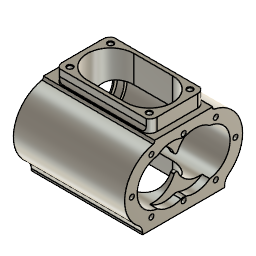
Body_ (Autodesk Fusion 360 design; units mm, degrees)
Autodesk Fusion 360 part; units mm, degrees
sketch "Sketch1" plane through (0, 0, 0) normal (1, 0, 0) x (0, 1, 0)
  circle A0 centre (-24, 0) radius 17.5
  arc A1 (-42.5, -37.3731) -> (-46.4362, -29.4214) centre (-52.5, -37.3731) ccw
  arc A2 (-31.4242, 36.2475) -> (-46.4362, -29.4214) centre (-24, 0) ccw
  arc A3 (-31.4242, 36.2475) -> (-30, 39.0239) centre (-31.8255, 38.2068) ccw
  line L0 (-30, 39.0239) -> (0, 39.0239)
  line L1 (0, 39.0239) -> (0, 0) construction
  line L2 (-42.5, -37.3731) -> (-42.5, -39.4214)
  line L3 (-42.5, -39.4214) -> (0, -39.4214)
  line L4 (0, 0) -> (0, -39.4214)
  line L5 (30, 39.0239) -> (0, 39.0239)
  arc A4 (30, 39.0239) -> (31.4242, 36.2475) centre (31.8255, 38.2068) ccw
  arc A5 (46.4362, -29.4214) -> (31.4242, 36.2475) centre (24, 0) ccw
  arc A6 (46.4362, -29.4214) -> (42.5, -37.3731) centre (52.5, -37.3731) ccw
  line L6 (42.5, -37.3731) -> (42.5, -39.4214)
  line L7 (42.5, -39.4214) -> (0, -39.4214)
  line L8 (0, 0) -> (0, -39.4214)
  circle A7 centre (24, 0) radius 17.5
  dimension "d1" = 35
  dimension "d2" = 24
  dimension "d3" = 2
  dimension "d4" = 37
  dimension "d5" = 10
  dimension "d6" = 10
  dimension "d7" = 42.5
  dimension "d8" = 30
  constraint horizontal L1.end A0.centre
  constraint tangent A1 A2
  constraint tangent A2 A3
  constraint horizontal L0
  constraint coincident L1.end L4.start
  constraint concentric A0 A2
  constraint vertical L2
  constraint perpendicular L2 L3
  constraint tangent A1 L2
  constraint vertical L4
  constraint vertical L1
  constraint symmetric A0 L1 A7
  constraint symmetric A1.start L1 A6.end
  constraint symmetric A1.end L1 A5.start
  constraint symmetric A1 L1 A6
  constraint symmetric A2.start L1 A4.end
  constraint symmetric A2 L1 A5
  constraint symmetric A3.end L1 L5.start
  constraint symmetric A3 L1 A4
  constraint symmetric L0.end L1 L5.end
  constraint symmetric L4.start L1 L8.start
  constraint symmetric L1 L2.end L6.end
  constraint symmetric L1 L3.end L4.end
  measures "d1" diameter of A0
  measures "d2" distance of L1.end A0.centre
  measures "d3" radius of A3
  measures "d4" radius of A2
  measures "d5" radius of A1
  measures "d6" vertical distance of A1.end L2.end
  measures "d7" distance of L2.end L3.end
  measures "d8" distance of A3.end L0.end
extrude "Extrude1" add sketch "Sketch1" along normal blind 115
sketch "Sketch2" plane through (115, 0, 0) normal (1, 0, 0) x (0, 1, 0)
  circle A0 centre (-24, 0) radius 17.5
  circle A1 centre (24, 0) radius 17.5
  arc A2 (46.4362, -29.4214) -> (31.4242, 36.2475) centre (24, 0) ccw
  arc A3 (30, 39.0239) -> (31.4242, 36.2475) centre (31.8255, 38.2068) ccw
  line L0 (30, 39.0239) -> (-30, 39.0239)
  arc A4 (-31.4242, 36.2475) -> (-30, 39.0239) centre (-31.8255, 38.2068) ccw
  arc A5 (-31.4242, 36.2475) -> (-46.4362, -29.4214) centre (-24, 0) ccw
  arc A6 (-42.5, -37.3731) -> (-46.4362, -29.4214) centre (-52.5, -37.3731) ccw
  line L1 (-42.5, -37.3731) -> (-42.5, -39.4214)
  line L2 (-42.5, -39.4214) -> (42.5, -39.4214)
  line L3 (42.5, -39.4214) -> (42.5, -37.3731)
  arc A7 (46.4362, -29.4214) -> (42.5, -37.3731) centre (52.5, -37.3731) ccw
  arc A8 (-1.8449, 9.2279) -> (1.8462, 9.2308) centre (0, 10) ccw
  arc A9 (1.8462, -9.2308) -> (-1.8461, -9.2308) centre (0, -10) ccw
  arc A10 (-1.8449, 9.2279) -> (-1.8461, -9.2308) centre (-24, 0) ccw
  arc A11 (1.8462, -9.2308) -> (1.8462, 9.2308) centre (24, 0) ccw
  dimension "d11" = 48
  dimension "d12" = 48
  dimension "d13" = 20
  dimension "d14" = 2
  dimension "d15" = 2
  constraint concentric A0 A10
  constraint concentric A1 A11
  constraint tangent A8 A11
  constraint tangent A9 A11
  measures "d11" diameter of A10
  measures "d12" diameter of A11
  measures "d13" vertical distance of A8.centre A9.centre
  measures "d14" radius of A9
  measures "d15" radius of A8
extrude "Extrude2" cut sketch "Sketch2" against normal blind 106.5 contours A8 A9 A10 A11
sketch "Sketch3" plane through (115, 0, 0) normal (1, 0, 0) x (0, 1, 0)
  arc A0 (1.8462, -9.2308) -> (-1.8461, -9.2308) centre (0, -10) ccw
  arc A1 (-1.8449, 9.2279) -> (-1.8461, -9.2308) centre (-24, 0) ccw
  arc A2 (-1.8449, 9.2279) -> (1.8462, 9.2308) centre (0, 10) ccw
  arc A3 (1.8462, -9.2308) -> (1.8462, 9.2308) centre (24, 0) ccw
  arc A4 (46.4362, -29.4214) -> (31.4242, 36.2475) centre (24, 0) ccw
  arc A5 (30, 39.0239) -> (31.4242, 36.2475) centre (31.8255, 38.2068) ccw
  line L0 (30, 39.0239) -> (-30, 39.0239)
  arc A6 (-31.4242, 36.2475) -> (-30, 39.0239) centre (-31.8255, 38.2068) ccw
  arc A7 (-31.4242, 36.2475) -> (-46.4362, -29.4214) centre (-24, 0) ccw
  arc A8 (-42.5, -37.3731) -> (-46.4362, -29.4214) centre (-52.5, -37.3731) ccw
  line L1 (-42.5, -37.3731) -> (-42.5, -39.4214)
  line L2 (-42.5, -39.4214) -> (42.5, -39.4214)
  line L3 (42.5, -39.4214) -> (42.5, -37.3731)
  arc A9 (46.4362, -29.4214) -> (42.5, -37.3731) centre (52.5, -37.3731) ccw
  line L4 (0, 0) -> (0, 67.4352) construction
  arc A10 (-2.5795, 27.2102) -> (-27, 23.8118) centre (-11.792, 3.9695) ccw
  arc A11 (-2.5795, 27.2102) -> (2.5795, 27.2102) centre (0, 33.7176) ccw
  arc A12 (27, 23.8118) -> (2.5795, 27.2102) centre (11.792, 3.9695) ccw
  dimension "d18" = 7
  dimension "d19" = 25
  dimension "d20" = 54
  constraint coincident L4.start origin
  constraint perpendicular L0 L4
  constraint coincident A1 A10.end
  constraint tangent A10 A11
  constraint tangent A11 A12
  constraint coincident A3 A12.start
  constraint equal A10 A12
  constraint symmetric L4 A10 A12
  constraint midpoint L4 A11.centre
  measures "d18" radius of A11
  measures "d19" radius of A10
  measures "d20" distance of A10.end A12.start
extrude "Extrude3" cut sketch "Sketch3" against normal blind 8 contours A1 A2 A3 A10 A11 A12
sketch "Sketch4" plane through (8.5, 0, 0) normal (1, 0, 0) x (0, 1, 0)
  circle A0 centre (-24, 0) radius 17.5
  circle A1 centre (24, 0) radius 17.5
  arc A2 (-1.8449, 9.2279) -> (-1.8461, -9.2308) centre (-24, 0) ccw
  arc A3 (1.8462, -9.2308) -> (-1.8461, -9.2308) centre (0, -10) ccw
  arc A4 (1.8462, -9.2308) -> (1.8462, 9.2308) centre (24, 0) ccw
  arc A5 (-1.8449, 9.2279) -> (1.8462, 9.2308) centre (0, 10) ccw
  circle A6 centre (-24, 0) radius 21
  circle A7 centre (24, 0) radius 21
  dimension "d23" = 42
  dimension "d24" = 42
  constraint concentric A0 A6
  constraint concentric A1 A7
  measures "d23" diameter of A6
  measures "d24" diameter of A7
extrude "Extrude4" cut sketch "Sketch4" against normal blind 7 contours A6 | A7
sketch "Sketch5" plane through (0, 0, 39.0239) normal (0, 0, 1) x (-1, 0, 0)
  line L0 (0, -30) -> (0, 30)
  line L1 (0, 30) -> (-115, 30)
  line L2 (-115, 30) -> (-115, -30)
  line L3 (-115, -30) -> (0, -30)
  line L4 (-10.5, -29) -> (-108.5, -29)
  line L5 (-108.5, -29) -> (-108.5, 29)
  line L6 (-108.5, 29) -> (-10.5, 29)
  line L7 (-10.5, 29) -> (-10.5, -29)
  line L8 (-10.5, -29) -> (-108.5, 29) construction
  line L9 (-108.5, -29) -> (-10.5, 29) construction
  point P0 (-59.5, 0)
  dimension "d27" = 10.5
  dimension "d28" = 58
  dimension "d29" = 98
  constraint horizontal L4
  constraint perpendicular L4 L5
  constraint parallel L4 L6
  constraint parallel L5 L7
  constraint coincident L8 P0
  constraint coincident L9 P0
  constraint midpoint L8 P0
  constraint horizontal origin P0
  measures "d27" distance of L0 L7
  measures "d28" distance of L4.start L6.end
  measures "d29" distance of L5.end L6.end
extrude "Extrude5" add sketch "Sketch5" along normal blind 13 contours L4 L5 L6 L7
fillet "Fillet1" radius 8 4 edges at (108.5, -29, 45.5239) (108.5, 29, 45.5239) (10.5, 29, 45.5239) (10.5, -29, 45.5239)
sketch "Sketch6" plane through (0, 0, 52.0239) normal (0, 0, 1) x (-1, 0, 0)
  arc A0 (-10.5, 21) -> (-18.5, 29) centre (-18.5, 21) ccw
  line L0 (-18.5, 29) -> (-100.5, 29)
  arc A1 (-100.5, 29) -> (-108.5, 21) centre (-100.5, 21) ccw
  line L1 (-108.5, 21) -> (-108.5, -21)
  arc A2 (-108.5, -21) -> (-100.5, -29) centre (-100.5, -21) ccw
  line L2 (-100.5, -29) -> (-18.5, -29)
  arc A3 (-18.5, -29) -> (-10.5, -21) centre (-18.5, -21) ccw
  line L3 (-10.5, -21) -> (-10.5, 21)
  line L4 (-39.5, 24) -> (-79.5, 24)
  arc A4 (-79.5, 24) -> (-79.5, -24) centre (-79.5, 0) ccw
  line L5 (-79.5, -24) -> (-39.5, -24)
  arc A5 (-39.5, -24) -> (-39.5, 24) centre (-39.5, 0) ccw
  line L6 (-39.5, 0) -> (-79.5, 0) construction
  point P0 (-59.5, 0)
  dimension "d34" = 24
  dimension "d35" = 40
  dimension "d36" = 29
  constraint tangent L4 A4
  constraint tangent A4 L5
  constraint parallel L4 L5
  constraint tangent L5 A5
  constraint tangent L4 A5
  constraint perpendicular L3 L6
  constraint midpoint L6 P0
  constraint horizontal origin P0
  measures "d34" radius of A4
  measures "d35" distance of L4.start L4.end
  measures "d36" distance of L1 A4.centre
extrude "Extrude6" cut sketch "Sketch6" against normal blind 100 contours L4 A4 L5 A5
sketch "Sketch7" plane through (108.5, 0, 0) normal (1, 0, 0) x (0, 1, 0)
  line L0 (21, 39.0239) -> (21, 52.0239)
  line L1 (21, 52.0239) -> (-21, 52.0239)
  line L2 (-21, 52.0239) -> (-21, 39.0239)
  line L3 (-21, 39.0239) -> (21, 39.0239)
  line L4 (-28, 52.0239) -> (-28, 45.0239)
  arc A0 (-29, 40.0239) -> (-28, 45.0239) centre (-41, 45.0239) ccw
  line L5 (-29, 52.0239) -> (-21, 52.0239)
  line L6 (-29, 52.0239) -> (-29, 39.0239)
  dimension "d39" = 1
  dimension "d40" = 1
  dimension "d41" = 7
  constraint vertical L4
  constraint tangent L4 A0
  constraint coincident L4.start L5
  constraint coincident A0.start L6
  measures "d39" distance of L4.start L5.start
  measures "d40" distance of A0.start L6.end
  measures "d41" distance of L4.start L4.end
extrude "Extrude7" cut sketch "Sketch7" against normal up to surface (98 mm away) contours L4 A0 L5 L6
mirror "Mirror1" about plane through (0, 0, 0) normal (0, 1, 0) of "Extrude7"
sketch "Sketch8" plane through (0, 0, 52.0239) normal (0, 0, 1) x (-1, 0, 0)
  line L0 (-104.373, -28) -> (-14.627, -28)
  arc A0 (-14.627, -28) -> (-10.5, -21) centre (-18.5, -21) ccw
  line L1 (-10.5, -21) -> (-10.5, 21)
  arc A1 (-10.5, 21) -> (-14.627, 28) centre (-18.5, 21) ccw
  line L2 (-14.627, 28) -> (-104.373, 28)
  arc A2 (-104.373, 28) -> (-108.5, 21) centre (-100.5, 21) ccw
  line L3 (-108.5, 21) -> (-108.5, -21)
  arc A3 (-108.5, -21) -> (-104.373, -28) centre (-100.5, -21) ccw
  line L4 (-79.5, 24) -> (-39.5, 24)
  arc A4 (-39.5, -24) -> (-39.5, 24) centre (-39.5, 0) ccw
  line L5 (-39.5, -24) -> (-79.5, -24)
  arc A5 (-79.5, 24) -> (-79.5, -24) centre (-79.5, 0) ccw
  circle A6 centre (-100.5, 21) radius 3
  circle A7 centre (-100.5, -21) radius 3
  circle A8 centre (-18.5, -21) radius 3
  circle A9 centre (-18.5, 21) radius 3
  dimension "d46" = 6
  dimension "d47" = 6
  dimension "d48" = 6
  dimension "d49" = 6
  constraint concentric A2 A6
  constraint concentric A3 A7
  constraint concentric A0 A8
  constraint concentric A1 A9
  measures "d46" diameter of A6
  measures "d47" diameter of A7
  measures "d48" diameter of A8
  measures "d49" diameter of A9
hole "Hole1" at (100.5, 21, 52.0239) at (100.5, -21, 52.0239) at (18.5, -21, 52.0239) at (18.5, 21, 52.0239) direction (0, 0, -1) diameter 5 depth 19 tip angle 180 countersink diameter 6 countersink angle 90
sketch "Sketch9" plane through (115, 0, 0) normal (1, 0, 0) x (0, 1, 0)
  arc A0 (27, 23.8118) -> (2.5795, 27.2102) centre (11.792, 3.9695) ccw
  arc A1 (1.8462, -9.2308) -> (27, 23.8118) centre (24, 0) ccw
  arc A2 (1.8462, -9.2308) -> (-1.8461, -9.2308) centre (0, -10) ccw
  arc A3 (-27, 23.8118) -> (-1.8461, -9.2308) centre (-24, 0) ccw
  arc A4 (-2.5795, 27.2102) -> (-27, 23.8118) centre (-11.792, 3.9695) ccw
  arc A5 (-2.5795, 27.2102) -> (2.5795, 27.2102) centre (0, 33.7176) ccw
  arc A6 (46.4362, -29.4214) -> (31.4242, 36.2475) centre (24, 0) ccw
  arc A7 (30, 39.0239) -> (31.4242, 36.2475) centre (31.8255, 38.2068) ccw
  line L0 (30, 39.0239) -> (-30, 39.0239)
  arc A8 (-31.4242, 36.2475) -> (-30, 39.0239) centre (-31.8255, 38.2068) ccw
  arc A9 (-31.4242, 36.2475) -> (-46.4362, -29.4214) centre (-24, 0) ccw
  arc A10 (-42.5, -37.3731) -> (-46.4362, -29.4214) centre (-52.5, -37.3731) ccw
  line L1 (-42.5, -37.3731) -> (-42.5, -39.4214)
  line L2 (-42.5, -39.4214) -> (42.5, -39.4214)
  line L3 (42.5, -39.4214) -> (42.5, -37.3731)
  arc A11 (46.4362, -29.4214) -> (42.5, -37.3731) centre (52.5, -37.3731) ccw
  circle A12 centre (-24, 0) radius 29.5 construction
  line L4 (0, 0) -> (0, 37.1626) construction
  point P0 (-33.2871, 28)
  point P1 (-53.5, 0)
  point P2 (-33.2871, -28)
  point P3 (0, -30)
  point P4 (0, 30)
  point P5 (33.2871, 28)
  point P6 (53.5, 0)
  point P7 (33.2871, -28)
  dimension "d55" = 59
  dimension "d56" = 28
  dimension "d57" = 30
  dimension "d58" = 30
  constraint concentric A3 A12
  constraint coincident A12 P0
  constraint coincident A12 P1
  constraint coincident A12 P2
  constraint coincident L4.start origin
  constraint vertical L4
  constraint horizontal L4.start P1
  constraint vertical L4.start P4
  constraint vertical P0 P2
  constraint vertical L4.start P3
  constraint symmetric P0 L4 P5
  constraint symmetric P1 L4 P6
  constraint symmetric P2 L4 P7
  measures "d55" diameter of A12
  measures "d56" vertical distance of A3.centre P0
  measures "d57" distance of L4.start P4
  measures "d58" distance of L4.start P3
hole "Hole2" at (115, 0, 30) at (115, -33.2871, 28) at (115, -53.5, 0) at (115, -33.2871, -28) at (115, 0, -30) at (115, 33.2871, -28) at (115, 53.5, 0) at (115, 33.2871, 28) direction (-1, 0, 0) diameter 5 depth 8 tip angle 118
mirror "Mirror2" about plane through (0, 0, 0) normal (0, 0, 1) of "Extrude3"
